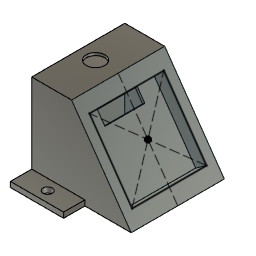
enclosure (Autodesk Fusion 360 design; units mm, degrees)
Autodesk Fusion 360 part; units mm, degrees
sketch "Sketch1" plane through (0, 0, 0) normal (0, 1, 0) x (1, 0, 0)
  line L0 (0, 0) -> (0, -32)
  line L1 (0, -32) -> (15, -32)
  line L2 (15, -32) -> (37.4066, 0)
  line L3 (0, 0) -> (37.4066, 0)
  dimension "d1" = 32
  dimension "d2" = 15
  dimension "d3" = 125
  constraint coincident L0.start L3.start
  constraint vertical L0
  constraint perpendicular L0 L1
  constraint perpendicular L0 L3
  measures "d1" distance of L0.start L0.end
  measures "d2" distance of L0.end L1.end
  measures "d3" angle of L1 L2
extrude "Extrude1" add sketch "Sketch1" along normal blind 35
sketch "Sketch3" plane through (25.1002, 0, 17.5754) normal (0.819152, 0, 0.573576) x (0, 1, 0)
  line L0 (0, 17.6092) -> (0, -21.4556)
  line L1 (0, -21.4556) -> (35, -21.4556)
  line L2 (35, -21.4556) -> (35, 17.6092)
  line L3 (35, 17.6092) -> (0, 17.6092)
  line L4 (17.5, 17.6092) -> (17.5, -21.4556) construction
  line L5 (31.5, -15.9232) -> (3.5, -15.9232)
  line L6 (3.5, -15.9232) -> (3.5, 12.0768)
  line L7 (3.5, 12.0768) -> (31.5, 12.0768)
  line L8 (31.5, 12.0768) -> (31.5, -15.9232)
  line L9 (31.5, -15.9232) -> (3.5, 12.0768) construction
  line L10 (3.5, -15.9232) -> (31.5, 12.0768) construction
  point P0 (17.5, -1.9232)
  dimension "d10" = 28
  dimension "d11" = 28
  constraint midpoint L3 L4.start
  constraint midpoint L1 L4.end
  constraint horizontal L5
  constraint perpendicular L5 L6
  constraint parallel L5 L7
  constraint parallel L6 L8
  constraint coincident L9 P0
  constraint coincident L10 P0
  constraint midpoint L4 P0
  measures "d10" distance of L6.end L7.end
  measures "d11" distance of L5.end L6.end
extrude "Extrude4" cut sketch "Sketch3" against normal blind 5 contours L5 L6 L7 L8
shell "Shell1" thickness 1 removed faces 1 at (12.4689, 11.6667, 0)
sketch "Sketch5" plane through (20.1853, 0, 14.1339) normal (-0.819152, 0, -0.573576) x (0, -1, 0)
  line L0 (-2.5, 13.0768) -> (-32.5, 13.0768)
  line L1 (-32.5, 13.0768) -> (-32.5, -16.9232)
  line L2 (-32.5, -16.9232) -> (-2.5, -16.9232)
  line L3 (-2.5, -16.9232) -> (-2.5, 13.0768)
  line L4 (-17.5, 13.0768) -> (-17.5, -16.9232) construction
  line L5 (-10, 11.0768) -> (-25, 11.0768)
  line L6 (-25, 11.0768) -> (-25, 6.0768)
  line L7 (-25, 6.0768) -> (-10, 6.0768)
  line L8 (-10, 6.0768) -> (-10, 11.0768)
  line L9 (-10, 11.0768) -> (-25, 6.0768) construction
  line L10 (-25, 11.0768) -> (-10, 6.0768) construction
  line L11 (-17.5, 13.0768) -> (-7.3236, 13.0768) construction
  point P0 (-17.5, 8.5768)
  dimension "d17" = 15
  dimension "d18" = 5
  dimension "d19" = 2
  constraint midpoint L0 L4.start
  constraint midpoint L2 L4.end
  constraint horizontal L5
  constraint perpendicular L5 L6
  constraint parallel L5 L7
  constraint parallel L6 L8
  constraint coincident L9 P0
  constraint coincident L10 P0
  constraint coincident L4 P0
  constraint coincident L0 L11.end
  constraint perpendicular L8 L11
  measures "d17" distance of L6.end L7.end
  measures "d18" distance of L5.end L6.end
  measures "d19" distance of L5 L11
extrude "Extrude5" cut sketch "Sketch5" against normal blind 10 contours L5 L6 L7 L8
sketch "Sketch6" plane through (0, 0, 32) normal (0, 0, 1) x (-1, 0, 0)
  line L0 (0, 0) -> (-15, 0)
  line L1 (-15, 0) -> (-15, -35)
  line L2 (-15, -35) -> (0, -35)
  line L3 (0, -35) -> (0, 0)
  line L4 (0, -17.5) -> (-15, -17.5) construction
  circle A0 centre (-6.5, -17.5) radius 3.5
  circle A1 centre (-6.5, -17.5) radius 5 construction
  dimension "d22" = 7
  dimension "d23" = 10
  dimension "d24" = 6.5
  constraint midpoint L3 L4.start
  constraint midpoint L1 L4.end
  constraint concentric A0 A1
  measures "d22" diameter of A0
  measures "d23" diameter of A1
  measures "d24" distance of L4.start A0.centre
extrude "Extrude6" cut sketch "Sketch6" against normal blind 5 contours A0
sketch "Sketch7" plane through (0, 35, 0) normal (0, 1, 0) x (-1, 0, 0)
  line L0 (0, 32) -> (-15, 32)
  line L1 (-15, 32) -> (-37.4066, 0)
  line L2 (-37.4066, 0) -> (0, 0)
  line L3 (0, 0) -> (0, 32)
  line L4 (0, 0) -> (-20, 0)
  line L5 (-20, 0) -> (-20, 2)
  line L6 (-20, 2) -> (0, 2)
  line L7 (0, 2) -> (0, 0)
  dimension "d27" = 20
  dimension "d28" = 2
  constraint horizontal L4
  constraint vertical L5
  constraint horizontal L6
  constraint vertical L7
  constraint coincident L2.end L3.start
  measures "d27" distance of L2.end L4.end
  measures "d28" distance of L2.end L6.end
extrude "Extrude7" add sketch "Sketch7" along normal blind 8 contours L2 L3 L4 L5 L6 L7
sketch "Sketch8" plane through (0, 0, 2) normal (0, 0, 1) x (-1, 0, 0)
  line L0 (0, -35) -> (-20, -35)
  line L1 (-20, -35) -> (-20, -43)
  line L2 (-20, -43) -> (0, -43)
  line L3 (0, -43) -> (0, -35)
  line L4 (-10, -43) -> (-10, -35) construction
  circle A0 centre (-10, -39) radius 2.8 construction
  circle A1 centre (-10, -39) radius 1.75
  dimension "d31" = 5.6
  dimension "d32" = 3.5
  constraint midpoint L2 L4.start
  constraint midpoint L0 L4.end
  constraint midpoint L4 A0.centre
  constraint concentric A0 A1
  measures "d31" diameter of A0
  measures "d32" diameter of A1
extrude "Extrude8" cut sketch "Sketch8" against normal blind 2 contours A1
sketch "Sketch9" plane through (0, 0, 0) normal (0, -1, 0) x (1, 0, 0)
  line L0 (15, 32) -> (0, 32)
  line L1 (0, 32) -> (0, 0)
  line L2 (0, 0) -> (37.4066, 0)
  line L3 (37.4066, 0) -> (15, 32)
  line L4 (0, 0) -> (20, 0)
  line L5 (20, 0) -> (20, 2)
  line L6 (20, 2) -> (0, 2)
  line L7 (0, 2) -> (0, 0)
  dimension "d35" = 20
  dimension "d36" = 2
  constraint horizontal L4
  constraint vertical L5
  constraint horizontal L6
  constraint vertical L7
  constraint coincident L1.end L2.start
  measures "d35" distance of L1.end L4.end
  measures "d36" distance of L1.end L6.end
extrude "Extrude9" add sketch "Sketch9" along normal blind 8 contours L1 L2 L4 L5 L6 L7
sketch "Sketch10" plane through (0, 0, 2) normal (0, 0, 1) x (-1, 0, 0)
  line L0 (-20, 0) -> (0, 0)
  line L1 (0, 0) -> (0, 8)
  line L2 (0, 8) -> (-20, 8)
  line L3 (-20, 8) -> (-20, 0)
  line L4 (-10, 8) -> (-10, 0) construction
  circle A0 centre (-10, 4) radius 1.75
  dimension "d39" = 3.5
  constraint midpoint L2 L4.start
  constraint midpoint L0 L4.end
  constraint midpoint L4 A0.centre
  measures "d39" diameter of A0
extrude "Extrude10" cut sketch "Sketch10" against normal blind 2 contours A0
